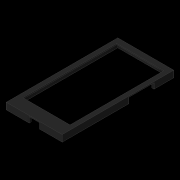
# Autodesk Inventor part: caseMain
Saved by Autodesk Inventor 2022 (Build 260153000, 153)
## iProperties
Created: 2022-09-01
Part Number: caseMain
Material: Generic
Document SubType Name: Modeling
Designer: Richy
Density: 1 g/cm^3
Appearance: Default
Author: Richy
Autodesk Inventor part; units mm, degrees
ref_plane "YZ Plane" through (0, 0, 0) normal (1, 0, 0) x (0, 1, 0)
ref_plane "XZ Plane" through (0, 0, 0) normal (0, 1, 0) x (-1, 0, 0)
ref_plane "XY Plane" through (0, 0, 0) normal (0, 0, 1) x (1, 0, 0)
sketch "Sketch1" plane through (0, 0, 0) normal (0, 1, 0) x (-1, 0, 0)
  line L0 (0, 0) -> (-76.2, 0)
  line L1 (-76.2, 0) -> (-76.2, -157.8)
  line L2 (-76.2, -157.8) -> (0, -157.8)
  line L3 (0, -157.8) -> (0, 0)
  line L4 (-76.2, -157.8) -> (-79.2, -157.8)
  line L5 (-79.2, -157.8) -> (-79.2, 0)
  line L6 (-79.2, 0) -> (-76.2, 0)
  line L7 (-76.2, 0) -> (-76.2, -157.8)
  line L8 (0, -157.8) -> (3, -157.8)
  line L9 (3, -157.8) -> (3, 0)
  line L10 (3, 0) -> (0, 0)
  line L11 (0, 0) -> (0, -157.8)
  line L12 (3, 0) -> (-79.2, 0)
  line L13 (-79.2, 0) -> (-79.2, 3)
  line L14 (-79.2, 3) -> (3, 3)
  line L15 (3, 3) -> (3, 0)
  line L16 (-30.6, 0) -> (-45.6, 0)
  line L17 (-45.6, 0) -> (-45.6, 3)
  line L18 (-45.6, 3) -> (-30.6, 3)
  line L19 (-30.6, 3) -> (-30.6, 0)
  line L20 (3, -157.8) -> (-79.2, -157.8)
  line L21 (-79.2, -157.8) -> (-79.2, -160.8)
  line L22 (-79.2, -160.8) -> (3, -160.8)
  line L23 (3, -160.8) -> (3, -157.8)
  dimension "d0" = 76.2
  dimension "d1" = 157.8
  dimension "d2" = 3
  dimension "d3" = 3
  dimension "d4" = 3
  dimension "d5" = 15
  dimension "d6" = 33.6
  dimension "d7" = 33.6
  dimension "d8" = 3
  constraints: 48 end point, 12 parallel, 6 horizontal, 6 perpendicular, 3 point on line
  measures "d0" distance of L1.end L2.end
  measures "d1" distance of L0.end L1.end
  measures "d2" distance between parallel lines of L3 L9
  measures "d3" distance between parallel lines of L1 L5
  measures "d4" distance between parallel lines of L12 L14
  measures "d5" distance between parallel lines of L17 L19
  measures "d6" distance between parallel lines of L15 L19
  measures "d7" distance between parallel lines of L13 L17
  measures "d8" distance of L20.end L21.end
extrude "Extrusion1" add sketch "Sketch1" along normal blind 8.2 contours L10 L9 L8 L3 | L0 L19 L14 L15 L10 | L8 L23 L22 L21 L4 L2 | L0 L6 L13 L14 L17 | L4 L5 L6 L1
sketch "Sketch6" plane through (0, 8.2, 0) normal (0, 1, 0) x (1, 0, 0)
  line L0 (79.2, -3) -> (79.2, 160.8) projected
  line L1 (-3, -3) -> (79.2, -3)
  line L2 (79.2, -3) -> (79.2, 15)
  line L3 (79.2, 15) -> (-3, 15)
  line L4 (-3, 15) -> (-3, -3)
  line L5 (-3, 160.8) -> (-3, -3) projected
  line L6 (-3, 160.8) -> (79.2, 160.8)
  line L7 (79.2, 160.8) -> (79.2, 152.8)
  line L8 (79.2, 152.8) -> (-3, 152.8)
  line L9 (-3, 152.8) -> (-3, 160.8)
  line L10 (-3, 15) -> (3.5, 15)
  line L11 (3.5, 15) -> (3.5, 152.8)
  line L12 (3.5, 152.8) -> (-3, 152.8)
  line L13 (-3, 152.8) -> (-3, 15)
  line L14 (79.2, 152.8) -> (72.7, 152.8)
  line L15 (72.7, 152.8) -> (72.7, 15)
  line L16 (72.7, 15) -> (79.2, 15)
  line L17 (79.2, 15) -> (79.2, 152.8)
  point P0 (0, 0)
  dimension "d22" = 18
  dimension "d23" = 8
  dimension "d24" = 6.5
  dimension "d25" = 6.5
  constraints: 32 end point, 8 parallel, 4 horizontal, 4 perpendicular, 4 point on line
  measures "d22" distance between parallel lines of L3 L1
  measures "d23" distance between parallel lines of L6 L8
  measures "d24" distance between parallel lines of L13 L11
  measures "d25" distance between parallel lines of L0 L15
extrude "Extrusion5" add sketch "Sketch6" along normal blind 1.5 contours L1 L4 L3 L0 | L3 L15 L8 L0 | L8 L5 L6 L0 | L5 L8 L11 L3
sketch "Sketch7" plane through (76.2, 0, -157.8) normal (-1, 0, 0) x (0, 0, 1)
  line L0 (0, 8.2) -> (157.8, 8.2) projected
  line L1 (0, 0) -> (157.8, 0) projected
  line L2 (26, 8.2) -> (63, 8.2)
  line L3 (63, 8.2) -> (63, 0)
  line L4 (63, 0) -> (26, 0)
  line L5 (26, 0) -> (26, 8.2)
  line L6 (0, 0) -> (0, 8.2) projected
  point P0 (26, 0)
  dimension "d28" = 37
  dimension "d29" = 26
  constraints: 8 end point, 2 parallel, 2 point on line, 1 horizontal, 1 perpendicular
  measures "d28" distance between parallel lines of L5 L3
  measures "d29" distance between parallel lines of L5 L6
extrude "Extrusion6" cut sketch "Sketch7" against normal blind 8 contours L0 L3 L1 L5
body "Solid1"
